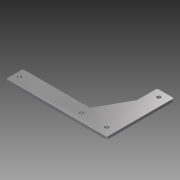
# Autodesk Inventor part: ZBedSupportPlate
Saved by Autodesk Inventor 2016 (Build 200138000, 138)
## iProperties
Category: Sheet Metal
Created: 2015-01-12
Part Number: ZBedSupportPlate
Material: Steel, Alloy
Document SubType Name: Modeling
Designer: Jack
Density: 7.73 g/cm^3
Appearance: Semi-Polished
Mass: 97.6406 g
Surface Area: 93.3834 cm^2
Volume: 12.6314 cm^3
Catalog Web Link: N/A
Author: Jack
Title: Z Bed Support
Autodesk Inventor part; units mm, degrees
ref_plane "YZ Plane" through (0, 0, 0) normal (1, 0, 0) x (0, 1, 0)
ref_plane "XZ Plane" through (0, 0, 0) normal (0, 1, 0) x (-1, 0, 0)
ref_plane "XY Plane" through (0, 0, 0) normal (0, 0, 1) x (1, 0, 0)
sketch "Sketch1" plane through (0, 0, 0) normal (0, 0, 1) x (1, 0, 0)
  line L0 (0, 0) -> (120, 0)
  line L1 (120, 0) -> (120, 80)
  line L2 (0, 0) -> (0, 20)
  line L3 (120, 80) -> (100, 80)
  line L4 (0, 20) -> (80, 20)
  line L5 (100, 80) -> (100, 56)
  line L6 (100, 56) -> (80, 20)
  dimension "d0" = 120
  dimension "d1" = 80
  dimension "d16" = 20
  dimension "d17" = 20
  dimension "d19" = 80
  dimension "d21" = 36
  constraints: 14 end point, 3 horizontal, 2 vertical, 1 perpendicular
  measures "d0" distance of L0.start L0.end
  measures "d1" distance of L0.end L1.end
  measures "d16" distance of L0.start L2.end
  measures "d17" distance of L1.end L3.end
  measures "d19" distance of L2.end L4.end
  measures "d21" vertical distance of L5.end L4.end
extrude "Extrusion1" add sketch "Sketch1" along normal blind 3.175
sketch "Sketch2" plane through (0, 0, 3.175) normal (0, 0, 1) x (1, 0, 0)
  line L0 (0, 0) -> (120, 0) projected
  line L1 (120, 0) -> (120, 80) projected
  circle A0 centre (6, 10) radius 2.25
  circle A1 centre (80, 10) radius 2.25
  circle A2 centre (110, 10) radius 2.25
  circle A3 centre (110, 72) radius 2.25
  line L2 (0, 20) -> (0, 0) projected
  point P0 (0, 15)
  dimension "d5" = 4.5
  dimension "d7" = 10
  dimension "d9" = 40
  dimension "d10" = 10
  dimension "d11" = 8
  dimension "d18" = 6
  constraints: 4 centre point, 3 equal radius, 2 horizontal alignment, 1 vertical alignment
  measures "d5" diameter of A3
  measures "d7" distance from line of L1 A2.centre
  measures "d9" distance from line of L1 A1.centre
  measures "d10" distance from line of L0 A2.centre
  measures "d11" vertical distance of L1.end A3.centre
  measures "d18" distance from line of L2 A0.centre
extrude "Extrusion2" cut sketch "Sketch2" against normal up to next
fillet "Fillet1" radius 2 3 edges at (120, 80, 1.5875) (0, 20, 1.5875) (100, 80, 1.5875)
fillet "Fillet2" radius 2 2 edges at (0, 0, 1.5875) (120, 0, 1.5875)
body "Solid1"
